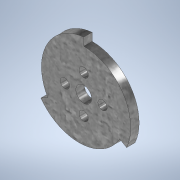
# Autodesk Inventor part: Weapon
Saved by Autodesk Inventor 2022 (Build 260153000, 153)
## iProperties
Created: 2022-08-11
Part Number: Weapon
Material: Steel
Document SubType Name: Modeling
Designer: Nick
Density: 7.85 g/cm^3
Appearance: Steel Galvanized
Mass: 170.357 g
Surface Area: 86.0172 cm^2
Volume: 21.7015 cm^3
Author: Nick
Autodesk Inventor part; units mm, degrees
ref_plane "YZ Plane" through (0, 0, 0) normal (1, 0, 0) x (0, 1, 0)
ref_plane "XZ Plane" through (0, 0, 0) normal (0, 1, 0) x (-1, 0, 0)
ref_plane "XY Plane" through (0, 0, 0) normal (0, 0, 1) x (1, 0, 0)
sketch "Sketch1" plane through (0, 0, 0) normal (0, 0, 1) x (1, 0, 0)
  circle A0 centre (0, 0) radius 37.5 construction
  circle A1 centre (0, 0) radius 31.5
  line L0 (0, 31.5) -> (0, 37.5)
  arc A2 (0, 37.5) -> (-27.2798, -15.75) centre (3.5675, 2.0597) ccw
  line L1 (0, 0) -> (-27.2798, -15.75) construction
  circle A3 centre (0, 0) radius 6
  dimension "d0" = 75
  dimension "d1" = 120
  dimension "d2" = 6
  dimension "d8" = 12
  constraints: 4 end point, 4 point on circle, 3 centre point, 3 coincident, 2 vertical alignment, 1 tangent, 1 vertical, 2 other
  measures "d1" angle of L0 L1
  measures "d2" distance of L0.start L0.end
  measures "d8" diameter of A3
extrude "Extrusion1" add sketch "Sketch1" along normal blind 6.35
pattern_circular "Circular Pattern1" count 3 over 360 about axis through (0, 0, 0) along (0, 0, 1) of "Extrusion1"
sketch "Sketch2" plane through (0, 0, 6.35) normal (0, 0, 1) x (1, 0, 0)
  circle A0 centre (0, 0) radius 14.25 construction
  point P0 (0, 14.25)
  dimension "d9" = 28.5
  constraints: 2 vertical alignment, 1 coincident, 2 other
hole "Hole1" at (0, 14.25, 6.35) direction (0, 0, -1) diameter 7 end through all clearance for "Flat Head Machine Screw" size "M6" standard "Ansi Metric M Profile"
pattern_circular "Circular Pattern2" count 4 over 360 about axis through (0, 0, 0) along (0, 0, 1) of "Hole1"
body "Solid1"
